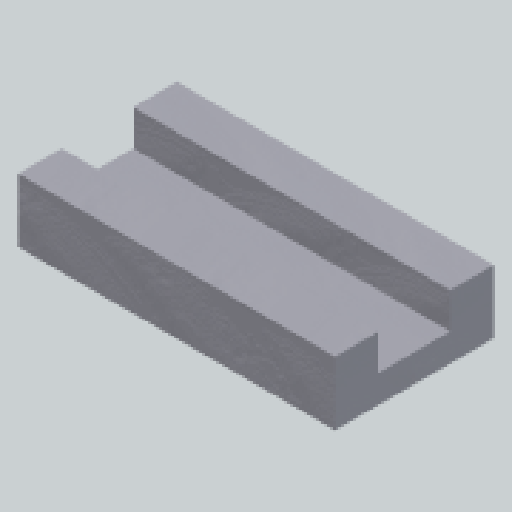
# Autodesk Inventor part: MGN9H
Saved by Autodesk Inventor 2023.2 (Build 272271000, 271)
## iProperties
Created: 2020-05-08
Part Number: MGN9H
Material: Stainless Steel AISI 440C, Welded
Document SubType Name: Modeling
Designer: Remo
Mass: 36.4135 g
Surface Area: 29.9017 cm^2
Volume: 4.66839 cm^3
Density: 7.8 g/cm^3
Appearance: Weld - Stainless Steel
Description: HIWIN MGN9H Linear Bearing Block
Author: Remo
Autodesk Inventor part; units mm, degrees
ref_plane "YZ Plane" through (0, 0, 0) normal (1, 0, 0) x (0, 1, 0)
ref_plane "XZ Plane" through (0, 0, 0) normal (0, 1, 0) x (-1, 0, 0)
ref_plane "XY Plane" through (0, 0, 0) normal (0, 0, 1) x (1, 0, 0)
sketch "Sketch1" plane through (0, 0, 0) normal (1, 0, 0) x (0, 1, 0)
  line L0 (-10, 4) -> (10, 4)
  line L1 (10, 4) -> (10, -4)
  line L2 (10, -4) -> (-10, -4)
  line L3 (-10, -4) -> (-10, 4)
  line L4 (-10, 4) -> (10, -4) construction
  line L5 (10, 4) -> (-10, -4) construction
  point P0 (0, 0)
  dimension "d0" = 8
  dimension "d1" = 20
  constraints: 12 end point, 2 equal length, 2 midpoint, 1 horizontal, 1 parallel
  measures "d0" distance of L0.end L1.end
  measures "d1" distance of L1.end L2.end
extrude "Extrusion1" add sketch "Sketch1" along normal blind 39.9
sketch "Sketch2" plane through (39.9, 0, 0) normal (1, 0, 0) x (0, 0, -1)
  line L0 (-4, 10) -> (-4, -10) projected
  line L1 (-4, 4.5) -> (0.5, 4.5)
  line L2 (0.5, 4.5) -> (0.5, -4.5)
  line L3 (0.5, -4.5) -> (-4, -4.5)
  line L4 (-4, -4.5) -> (-4, 4.5)
  point P0 (0, 0)
  dimension "d4" = 9
  dimension "d5" = 4.5
  dimension "d6" = 4.5
  constraints: 8 end point, 2 parallel, 1 horizontal, 1 perpendicular, 1 point on line
  measures "d4" distance between parallel lines of L3 L1
  measures "d5" distance from line of L1 point (0, 0)
  measures "d6" distance of L1.start L1.end
extrude "Extrusion2" cut sketch "Sketch2" against normal blind 39.9
sketch "Sketch3" plane through (0, -10, -4) normal (0, 0, -1) x (-1, 0, 0)
  line L0 (0, 20) -> (0, 0) projected
  line L1 (0, 20) -> (-39.9, 20) projected
  line L2 (-39.9, 0) -> (-39.9, 20) projected
  line L3 (0, 0) -> (-39.9, 0) projected
  point P0 (0, 10)
  point P1 (-27.95, 17.5)
  point P2 (-27.95, 2.5)
  point P3 (-11.95, 2.5)
  point P4 (-11.95, 17.5)
  dimension "d9" = 16
  dimension "d10" = 39.9
  dimension "d11" = 11.95
  dimension "d12" = 15
  dimension "d13" = 7.5
  constraints: 2 horizontal alignment, 2 vertical alignment
  measures "d9" distance of point (-11.95, 17.5) point (-27.95, 17.5)
  measures "d10" distance of L0.start L1.end
  measures "d11" distance from line of L0 point (-11.95, 17.5)
  measures "d12" distance of point (-11.95, 2.5) point (-11.95, 17.5)
  measures "d13" vertical distance of point (-11.95, 2.5) point (0, 10)
hole "Hole1" at (27.95, 7.5, -4) at (27.95, -7.5, -4) at (11.95, -7.5, -4) at (11.95, 7.5, -4) direction (0, 0, 1) diameter 2.459 depth 5 tip angle 118 thread size "M3x0.5" class "6H" standard "ISO Metric profile"
equation "\"d5\" = 0.5 * d4"
equation "\"d11\" = 0.5 * d10 - 0.5 * d9"
equation "\"d13\" = 0.5 * d12"
body "Solid1"
